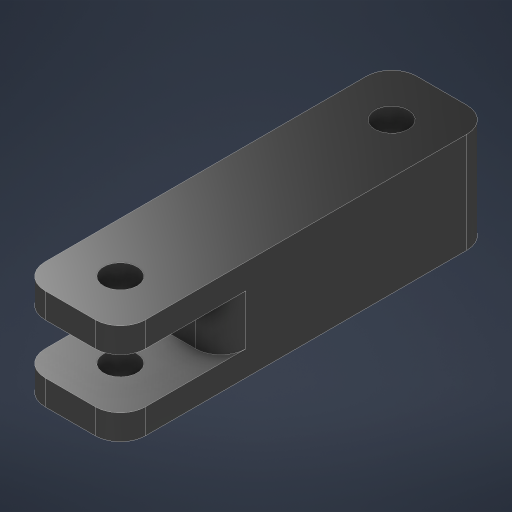
# Autodesk Inventor part: wing bar v2
Saved by Autodesk Inventor 2024 (Build 280153000, 153)
## iProperties
Created: 2023-12-25
Part Number: wing bar v2
Material: Generic
Document SubType Name: Modeling
Designer: elite
Density: 1 g/cm^3
Appearance: Glossy - Black
Author: elite
Autodesk Inventor part; units mm, degrees
ref_plane "YZ Plane" through (0, 0, 0) normal (1, 0, 0) x (0, 1, 0)
ref_plane "XZ Plane" through (0, 0, 0) normal (0, 1, 0) x (-1, 0, 0)
ref_plane "XY Plane" through (0, 0, 0) normal (0, 0, 1) x (1, 0, 0)
sketch "Sketch1" plane through (0, 0, 0) normal (1, 0, 0) x (0, 1, 0)
  line L0 (0, 0) -> (6.35, 0)
  line L1 (6.35, 0) -> (6.35, 12.7)
  line L2 (0, 0) -> (0, 12.7)
  line L3 (0, 12.7) -> (-3.175, 12.7)
  line L4 (-3.175, 12.7) -> (-3.175, -34.29)
  line L5 (6.35, 12.7) -> (9.525, 12.7)
  line L6 (9.525, 12.7) -> (9.525, -34.29)
  line L7 (9.525, -34.29) -> (-3.175, -34.29)
  dimension "d0" = 6.35
  dimension "d1" = 12.7
  dimension "d2" = 3.175
  dimension "d3" = 46.99
  dimension "d4" = 3.175
  constraints: 16 end point, 4 horizontal, 3 perpendicular, 1 vertical
  measures "d0" distance of L0.start L0.end
  measures "d1" distance of L0.end L1.end
  measures "d2" distance of L2.end L3.end
  measures "d3" distance of L3.end L4.end
  measures "d4" distance of L1.end L5.end
extrude "Extrusion1" add sketch "Sketch1" along normal blind 12.7
sketch "Sketch2" plane through (0, 9.525, 12.7) normal (0, 1, 0) x (1, 0, 0)
  line L0 (12.7, 0) -> (12.7, 46.99) projected
  line L1 (0, 12.7) -> (12.7, 0)
  circle A0 centre (6.35, 6.35) radius 2.1082
  dimension "d7" = 4.2164
  constraints: 2 end point, 1 centre point, 1 midpoint
  measures "d7" diameter of A0
extrude "Extrusion2" cut sketch "Sketch2" against normal blind 41.275
sketch "Sketch3" plane through (0, 9.525, 12.7) normal (0, 1, 0) x (1, 0, 0)
  line L0 (12.7, 0) -> (12.7, 46.99) projected
  line L1 (12.7, 46.99) -> (12.7, 34.29)
  line L2 (0, 0) -> (0, 46.99) projected
  line L3 (12.7, 34.29) -> (0, 46.99)
  circle A0 centre (6.35, 40.64) radius 2.1082
  point P0 (0, 12.7)
  dimension "d10" = 12.7
  dimension "d11" = 4.2164
  constraints: 4 end point, 1 centre point, 1 midpoint, 1 point on line
  measures "d10" distance of L0.end L1.end
  measures "d11" diameter of A0
extrude "Extrusion3" cut sketch "Sketch3" against normal blind 33.3375
fillet "Fillet1" radius 3.175 8 edges at (12.7, 3.175, -34.29) (0, 3.175, -34.29) (0, 7.9375, 12.7) (0, 3.175, 0) (12.7, 7.9375, 12.7) (12.7, 3.175, 0) (12.7, -1.5875, 12.7) (0, -1.5875, 12.7)
body "Solid1"
